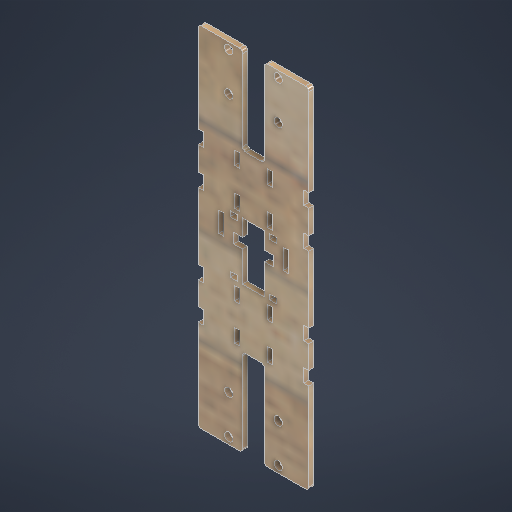
# Autodesk Inventor part: main_frame
Saved by Autodesk Inventor 2025.3 (Build 293356030, 356C)
## iProperties
Created: 2025-09-03
Part Number: main_frame
Material: 木材 (楓木)
Document SubType Name: Modeling
Designer: 陳泓任
Density: 0.67 g/cm^3
Appearance: 天然楓木 - 深色亮面處理
Author: 陳泓任
Autodesk Inventor part; units mm, degrees
ref_plane "YZ Plane" through (0, 0, 0) normal (1, 0, 0) x (0, 1, 0)
ref_plane "XZ Plane" through (0, 0, 0) normal (0, 1, 0) x (-1, 0, 0)
ref_plane "XY Plane" through (0, 0, 0) normal (0, 0, 1) x (1, 0, 0)
sketch "草圖1" plane through (0, 0, 0) normal (0, 0, 1) x (1, 0, 0)
  line L0 (-33, -104) -> (33, 104) construction
  line L1 (33, -104) -> (-33, 104) construction
  line L2 (0, 128.5379) -> (0, -160.5456) construction
  circle A0 centre (-14.75, 100) radius 2.5
  circle A1 centre (14.75, 100) radius 2.5
  circle A2 centre (14.75, 77) radius 2.5
  circle A3 centre (-14.75, 77) radius 2.5
  line L3 (-33, 49.8787) -> (-30, 49.8787)
  line L4 (-30, 49.8787) -> (-30, 41.8787)
  line L5 (-30, 41.8787) -> (-33, 41.8787)
  line L6 (-33, 102) -> (-33, 49.8787)
  line L7 (-11.2, 49.8787) -> (-8.2, 49.8787)
  line L8 (-8.2, 49.8787) -> (-8.2, 41.8787)
  line L9 (-8.2, 41.8787) -> (-11.2, 41.8787)
  line L10 (-11.2, 41.8787) -> (-11.2, 49.8787)
  line L11 (33, 49.8787) -> (30, 49.8787)
  line L12 (30, 49.8787) -> (30, 41.8787)
  line L13 (30, 41.8787) -> (33, 41.8787)
  line L14 (11.2, 49.8787) -> (8.2, 49.8787)
  line L15 (8.2, 49.8787) -> (8.2, 41.8787)
  line L16 (8.2, 41.8787) -> (11.2, 41.8787)
  line L17 (11.2, 41.8787) -> (11.2, 49.8787)
  line L18 (33, 49.8787) -> (33, 102)
  line L19 (-33, 41.8787) -> (-33, 27.6686)
  line L20 (33, 27.6686) -> (33, 41.8787)
  line L21 (-4.5, 52) -> (4.5, 52)
  line L22 (6.5, 54) -> (6.5, 102)
  line L23 (-6.5, 102) -> (-6.5, 54)
  line L24 (-6.5, 52) -> (6.5, 104) construction
  line L25 (6.5, 52) -> (-6.5, 104) construction
  line L26 (31, 104) -> (8.5, 104)
  line L27 (-8.5, 104) -> (-31, 104)
  arc A4 (-6.5, 102) -> (-8.5, 104) centre (-8.5, 102) ccw
  arc A5 (8.5, 104) -> (6.5, 102) centre (8.5, 102) ccw
  arc A6 (-6.5, 54) -> (-4.5, 52) centre (-4.5, 54) ccw
  arc A7 (4.5, 52) -> (6.5, 54) centre (4.5, 54) ccw
  arc A8 (-31, 104) -> (-33, 102) centre (-31, 102) ccw
  arc A9 (33, 102) -> (31, 104) centre (31, 102) ccw
  line L28 (-82.8249, 0) -> (86.4934, 0) construction
  circle A10 centre (-14.75, -100) radius 2.5
  circle A11 centre (14.75, -100) radius 2.5
  circle A12 centre (14.75, -77) radius 2.5
  circle A13 centre (-14.75, -77) radius 2.5
  line L29 (-33, -49.8787) -> (-30, -49.8787)
  line L30 (-30, -49.8787) -> (-30, -41.8787)
  line L31 (-30, -41.8787) -> (-33, -41.8787)
  line L32 (-33, -102) -> (-33, -49.8787)
  line L33 (-11.2, -49.8787) -> (-8.2, -49.8787)
  line L34 (-8.2, -49.8787) -> (-8.2, -41.8787)
  line L35 (-8.2, -41.8787) -> (-11.2, -41.8787)
  line L36 (-11.2, -41.8787) -> (-11.2, -49.8787)
  line L37 (33, -49.8787) -> (30, -49.8787)
  line L38 (30, -49.8787) -> (30, -41.8787)
  line L39 (30, -41.8787) -> (33, -41.8787)
  line L40 (8.2, -41.8787) -> (11.2, -41.8787)
  line L41 (11.2, -41.8787) -> (11.2, -49.8787)
  line L42 (8.2, -49.8787) -> (8.2, -41.8787)
  line L43 (11.2, -49.8787) -> (8.2, -49.8787)
  line L44 (33, -49.8787) -> (33, -102)
  line L45 (8.2, -28.1) -> (8.2, -20.1)
  line L46 (8.2, -20.1) -> (11.2, -20.1)
  line L47 (11.2, -28.1) -> (8.2, -28.1)
  line L48 (11.2, -20.1) -> (11.2, -28.1)
  line L49 (30, -28.1) -> (30, -20.1)
  line L50 (30, -20.1) -> (33, -20.1)
  line L51 (33, -28.1) -> (30, -28.1)
  line L52 (-8.2, -28.1) -> (-8.2, -20.1)
  line L53 (-8.2, -20.1) -> (-11.2, -20.1)
  line L54 (-11.2, -28.1) -> (-8.2, -28.1)
  line L55 (-11.2, -20.1) -> (-11.2, -28.1)
  line L56 (-30, -28.1) -> (-30, -20.1)
  line L57 (-33, -28.1) -> (-30, -28.1)
  line L58 (-30, -20.1) -> (-33, -20.1)
  line L59 (-33, -41.8787) -> (-33, -28.1)
  line L60 (33, -28.1) -> (33, -41.8787)
  line L61 (-4.5, -52) -> (4.5, -52)
  line L62 (6.5, -54) -> (6.5, -102)
  line L63 (-6.5, -102) -> (-6.5, -54)
  line L64 (-6.5, -52) -> (6.5, -104) construction
  line L65 (6.5, -52) -> (-6.5, -104) construction
  line L66 (31, -104) -> (8.5, -104)
  line L67 (-8.5, -104) -> (-31, -104)
  arc A14 (-8.5, -104) -> (-6.5, -102) centre (-8.5, -102) ccw
  arc A15 (6.5, -102) -> (8.5, -104) centre (8.5, -102) ccw
  arc A16 (-4.5, -52) -> (-6.5, -54) centre (-4.5, -54) ccw
  arc A17 (6.5, -54) -> (4.5, -52) centre (4.5, -54) ccw
  arc A18 (-33, -102) -> (-31, -104) centre (-31, -102) ccw
  arc A19 (31, -104) -> (33, -102) centre (31, -102) ccw
  line L68 (-31, -104) -> (-8.5, -104)
  line L69 (8.5, -104) -> (31, -104)
  line L70 (-6.65, -17.1) -> (6.65, -17.1)
  line L71 (6.65, 17.1) -> (-6.65, 17.1)
  line L72 (-6.65, -17.1) -> (6.65, 17.1) construction
  line L73 (6.65, -17.1) -> (-6.65, 17.1) construction
  line L74 (11.85, 1.05) -> (11.85, 7.05)
  line L75 (-11.85, 7.05) -> (-11.85, 1.05)
  line L76 (-11.85, 1.05) -> (11.85, 7.05) construction
  line L77 (11.85, 1.05) -> (-11.85, 7.05) construction
  line L78 (-6.65, 17.1) -> (-6.65, 7.05)
  line L79 (-6.65, 1.05) -> (-6.65, -17.1)
  line L80 (6.65, -17.1) -> (6.65, 1.05)
  line L81 (6.65, 7.05) -> (6.65, 17.1)
  line L82 (11.85, 7.05) -> (6.65, 7.05)
  line L83 (6.65, 1.05) -> (11.85, 1.05)
  line L84 (-11.85, 1.05) -> (-6.65, 1.05)
  line L85 (-6.65, 7.05) -> (-11.85, 7.05)
  line L86 (-33, -28.1) -> (-33, -41.8787)
  line L87 (-33, -49.8787) -> (-33, -102)
  line L88 (33, -102) -> (33, -49.8787)
  line L89 (33, -41.8787) -> (33, -28.1)
  line L90 (-11.2, -41.8787) -> (-8.2, -49.8787) construction
  line L91 (-8.2, -41.8787) -> (-11.2, -49.8787) construction
  line L92 (-13.3213, -39.7574) -> (-6.0787, -39.7574) construction
  line L93 (-6.0787, -39.7574) -> (-6.0787, -52) construction
  line L94 (-6.0787, -52) -> (-13.3213, -52) construction
  line L95 (-13.3213, -52) -> (-13.3213, -39.7574) construction
  line L96 (-8.2, -41.8787) -> (-6.0787, -39.7574) construction
  circle A20 centre (-6.65, 17.1) radius 3 construction
  line L97 (-11.2, 27.6686) -> (-8.2, 27.6686)
  line L98 (-8.2, 27.6686) -> (-8.2, 19.6686)
  line L99 (-8.2, 19.6686) -> (-11.2, 19.6686)
  line L100 (-11.2, 19.6686) -> (-11.2, 27.6686)
  line L101 (-33, 27.6686) -> (-30, 27.6686)
  line L102 (-30, 27.6686) -> (-30, 19.6686)
  line L103 (-30, 19.6686) -> (-33, 19.6686)
  line L104 (11.2, 27.6686) -> (8.2, 27.6686)
  line L105 (8.2, 27.6686) -> (8.2, 19.6686)
  line L106 (8.2, 19.6686) -> (11.2, 19.6686)
  line L107 (11.2, 19.6686) -> (11.2, 27.6686)
  line L108 (33, 27.6686) -> (30, 27.6686)
  line L109 (30, 27.6686) -> (30, 19.6686)
  line L110 (30, 19.6686) -> (33, 19.6686)
  line L111 (-33, 19.6686) -> (-33, -20.1)
  line L112 (33, 19.6686) -> (33, -20.1)
  line L113 (-9.65, -17.1) -> (-13.95, -17.1) construction
  line L114 (-13.95, -17.1) -> (-13.95, -14.1) construction
  line L115 (-13.95, -14.1) -> (-9.65, -14.1) construction
  line L116 (-9.65, -14.1) -> (-9.65, -17.1) construction
  line L117 (-16.95, -20.1) -> (-6.65, -20.1) construction
  line L118 (-6.65, -20.1) -> (-6.65, -11.1) construction
  line L119 (-6.65, -11.1) -> (-16.95, -11.1) construction
  line L120 (-16.95, -11.1) -> (-16.95, -20.1) construction
  point P0 (0, 0)
  point P1 (0, 86.5078)
  point P2 (0, 78)
  point P3 (0, -86.5078)
  point P4 (0, -78)
  point P5 (0, 4.05)
  point P6 (11.85, 4.05)
  dimension "d56" = 6
  dimension "d0" = 66
  dimension "d1" = 208
  dimension "d6" = 5
  dimension "d8" = 29.5
  dimension "d9" = 23
  dimension "d10" = 3
  dimension "d11" = 8
  dimension "d13" = 3
  dimension "d14" = 18.8
  dimension "d22" = 13
  dimension "d23" = 4
  dimension "d24" = 2
  dimension "d25" = 2
  dimension "d26" = 34.2
  dimension "d27" = 13.3
  dimension "d28" = 6
  dimension "d30" = 23.7
  dimension "d31" = 10.05
  dimension "d53" = 3
  dimension "d54" = 52
  dimension "d57" = 3
  dimension "d58" = 3
  dimension "d71" = 4.3
  dimension "d72" = 3
  dimension "d73" = 3
  dimension "d74" = 3
  constraints: 242 end point, 60 symmetric about line, 42 parallel, 29 point on line, 24 point on circle, 22 perpendicular, 20 centre point, 16 collinear, 15 horizontal, 12 tangent, 11 equal length, 9 midpoint, 7 equal radius, 4 vertical, 1 coincident, 1 vertical alignment, 21 other
  measures "d0" distance of L0.end L1.end
  measures "d1" distance of L1.start L0.end
  measures "d6" diameter of A0
  measures "d8" distance of A2.centre A3.centre
  measures "d9" distance of A1.centre A2.centre
  measures "d10" distance of L4.end L5.end
  measures "d11" distance of L3.end L4.end
  measures "d13" distance of L7.start L7.end
  measures "d14" distance between parallel lines of L4 L10
  measures "d22" distance of L24.start L25.start
  measures "d23" distance from line of A0.centre L27
  measures "d24" radius of A4
  measures "d25" radius of A8
  measures "d26" distance of L70.end L71.start
  measures "d27" distance of L71.start L71.end
  measures "d28" distance of L74.start L74.end
  measures "d30" distance from line of point (11.85, 4.05) L75
  measures "d31" distance between parallel lines of L85 L71
  measures "d53" distance of L35.start L92.end
  measures "d54" distance between parallel lines of L27 L21
  measures "d57" distance of L97.start L97.end
  measures "d58" distance of L19.end L101.end
  measures "d71" distance of L114.end L115.end
  measures "d72" distance between parallel lines of L79 L116
  measures "d73" distance of L113.end L114.end
  measures "d74" distance between parallel lines of L113 L117
extrude "擠出1" add sketch "草圖1" along normal blind 3
sketch "草圖3" plane through (0, 0, 3) normal (0, 0, 1) x (1, 0, 0)
  line L0 (-88.1264, 0) -> (75.7938, 0)
  line L1 (0, 123.8394) -> (0, -129.4918)
  point P0 (0, 0)
  constraints: 4 end point, 2 point on line, 1 horizontal, 1 perpendicular
sketch "草圖5" plane through (0, 0, 3) normal (0, 0, 1) x (1, 0, 0)
  line L0 (-9.65, -17.1) -> (-13.95, -17.1)
  line L1 (-13.95, -17.1) -> (-13.95, -14.1)
  line L2 (-13.95, -14.1) -> (-9.65, -14.1)
  line L3 (-9.65, -14.1) -> (-9.65, -17.1)
  line L4 (6.65, -17.1) -> (-6.65, -17.1) projected
  line L5 (-6.65, -17.1) -> (-6.65, 1.05) projected
  line L6 (-9.65, 14.1) -> (-13.95, 14.1)
  line L7 (-13.95, 14.1) -> (-13.95, 17.1)
  line L8 (-13.95, 17.1) -> (-9.65, 17.1)
  line L9 (-9.65, 17.1) -> (-9.65, 14.1)
  line L10 (-6.65, 17.1) -> (6.65, 17.1) projected
  line L11 (-6.65, 7.05) -> (-6.65, 17.1) projected
  line L12 (0, 31.1544) -> (0, -25.4134)
  line L13 (9.65, -17.1) -> (13.95, -17.1)
  line L14 (13.95, -17.1) -> (13.95, -14.1)
  line L15 (13.95, -14.1) -> (9.65, -14.1)
  line L16 (9.65, -14.1) -> (9.65, -17.1)
  line L17 (13.95, 17.1) -> (9.65, 17.1)
  line L18 (13.95, 14.1) -> (13.95, 17.1)
  line L19 (9.65, 14.1) -> (13.95, 14.1)
  line L20 (9.65, 17.1) -> (9.65, 14.1)
  line L21 (-17.65, 2.1) -> (-20.65, 2.1)
  line L22 (-20.65, 2.1) -> (-20.65, 14.1)
  line L23 (-20.65, 14.1) -> (-17.65, 14.1)
  line L24 (-17.65, 14.1) -> (-17.65, 2.1)
  line L25 (17.65, 2.1) -> (20.65, 2.1)
  line L26 (20.65, 2.1) -> (20.65, 14.1)
  line L27 (20.65, 14.1) -> (17.65, 14.1)
  line L28 (17.65, 14.1) -> (17.65, 2.1)
  point P0 (0, 0)
  dimension "d60" = 4.3
  dimension "d61" = 3
  dimension "d62" = 3
  dimension "d63" = 4.3
  dimension "d64" = 3
  dimension "d65" = 3
  dimension "d66" = 3
  dimension "d67" = 12
  dimension "d68" = 11
  constraints: 50 end point, 12 symmetric about line, 6 parallel, 3 collinear, 3 horizontal, 3 perpendicular, 1 point on line, 1 vertical
  measures "d60" distance of L0.start L0.end
  measures "d61" distance between parallel lines of L3 L5
  measures "d62" distance of L0.end L1.end
  measures "d63" distance of L6.start L7.start
  measures "d64" distance of L7.start L8.start
  measures "d65" distance between parallel lines of L9 L11
  measures "d66" distance of L22.end L23.end
  measures "d67" distance of L23.end L21.start
  measures "d68" distance between parallel lines of L5 L24
extrude "擠出4" cut sketch "草圖5" against normal up to next
